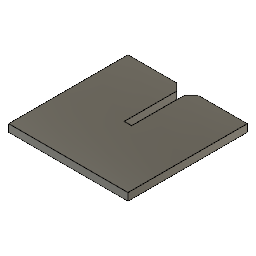
laser cutter parametric demo v2 (Autodesk Fusion 360 design; units mm, degrees)
Autodesk Fusion 360 part; units mm, degrees
sketch "Sketch1" plane through (0, 0, 0) normal (0, 0, 1) x (1, 0, 0)
  line L0 (0, 0) -> (50, 0)
  line L1 (50, 0) -> (50, 50)
  line L2 (50, 50) -> (0, 50)
  line L3 (0, 50) -> (0, 0)
  line L4 (25, 59.9444) -> (25, -10) construction
  line L5 (-9.9209, 25) -> (60, 25) construction
  line L6 (23.4218, 51.9444) -> (26.5218, 51.9444)
  line L7 (26.5218, 51.9444) -> (26.5218, 25)
  line L8 (26.5218, 25) -> (23.4218, 25)
  line L9 (23.4218, 25) -> (23.4218, 51.9444)
  dimension "d4" = 3.1
extrude "Extrude1" add sketch "Sketch1" along normal blind 3.2 contours L0 L1 L2 L3 L7 L8 L9
chamfer "Chamfer1" distance 3 angle 45 2 edges at (26.5218, 50, 1.6) (23.4218, 50, 1.6)
equation "material_thickness = 3.2 mm" comment "Real measured thickness of my plywood"
equation "laser_kerf = 0.1 mm" comment "Extra material removed for a given setting"
equation "chamfer_amount = 3 mm" comment "How much to round off each slot"
equation "d4 = material_thickness - laser_kerf"
equation "d5 = material_thickness"
equation "d7 = chamfer_amount"
